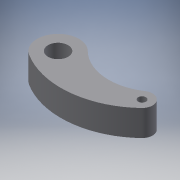
# Autodesk Inventor part: slider_link_p4
Saved by Autodesk Inventor 2017 (Build 210142000, 142)
## iProperties
Created: 2018-02-05
Part Number: slider_link_p4
Material: Generic
Document SubType Name: Modeling
Designer: Nic
Density: 1 g/cm^3
Appearance: Default
Author: Nic
Autodesk Inventor part; units mm, degrees
ref_plane "YZ Plane" through (0, 0, 0) normal (1, 0, 0) x (0, 1, 0)
ref_plane "XZ Plane" through (0, 0, 0) normal (0, 1, 0) x (-1, 0, 0)
ref_plane "XY Plane" through (0, 0, 0) normal (0, 0, 1) x (1, 0, 0)
sketch "Sketch1" plane through (0, 0, 0) normal (0, 0, 1) x (1, 0, 0)
  circle A0 centre (0, 0) radius 2.4
  arc A1 (21.7188, -1.8155) -> (18.6153, 2.0815) centre (20, 0) ccw
  arc A2 (3.5202, 3.5508) -> (-2.6562, -4.2361) centre (0, 0) ccw
  circle A3 centre (20, 0) radius 0.925
  arc A4 (-2.6562, -4.2361) -> (21.7188, -1.8155) centre (7.9688, 12.7082) ccw
  arc A5 (3.5202, 3.5508) -> (18.6153, 2.0815) centre (11.9688, 12.0727) ccw
  dimension "d0" = 4.8
  dimension "d3" = 2.5
  dimension "d6" = 5
  dimension "d7" = 20
  dimension "d8" = 1.85
  dimension "d9" = 20
  dimension "d10" = 12
  constraints: 8 point on circle, 6 centre point, 4 tangent, 2 coincident, 1 concentric, 1 horizontal alignment
  measures "d0" diameter of A0
  measures "d3" radius of A1
  measures "d6" radius of A2
  measures "d7" distance of A1.centre point (0, 0)
  measures "d8" diameter of A3
  measures "d9" radius of A4
  measures "d10" radius of A5
extrude "Extrusion1" add sketch "Sketch1" along normal blind 6.2
body "Solid1"
